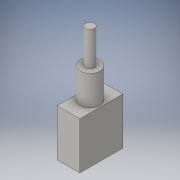
# Autodesk Inventor part: Switch
Saved by Autodesk Inventor 2016 (Build 200138000, 138)
## iProperties
Created: 2016-10-06
Part Number: Switch
Material: Generic
Document SubType Name: Modeling
Designer: sheehm
Density: 1 g/cm^3
Appearance: Default
Author: sheehm
Autodesk Inventor part; units mm, degrees
ref_plane "YZ Plane" through (0, 0, 0) normal (1, 0, 0) x (0, 1, 0)
ref_plane "XZ Plane" through (0, 0, 0) normal (0, 1, 0) x (-1, 0, 0)
ref_plane "XY Plane" through (0, 0, 0) normal (0, 0, 1) x (1, 0, 0)
sketch "Sketch1" plane through (0, 0, 0) normal (0, 1, 0) x (-1, 0, 0)
  line L0 (6.4234, 8.5987) -> (-0.2766, 8.5987)
  line L1 (-0.2766, 8.5987) -> (-0.2766, -4.1013)
  line L2 (-0.2766, -4.1013) -> (6.4234, -4.1013)
  line L3 (6.4234, -4.1013) -> (6.4234, 8.5987)
  point P0 (0, 0)
  dimension "d0" = 6.7
  dimension "d1" = 12.7
  constraints: 8 end point, 2 parallel, 1 horizontal, 1 perpendicular
  measures "d0" distance of L2.end L1.end
  measures "d1" distance of L1.end L0.end
extrude "Extrusion1" add sketch "Sketch1" along normal blind 13.9
sketch "Sketch2" plane through (0, 13.9, 0) normal (0, 1, 0) x (1, 0, 0)
  circle A0 centre (-3.0734, -2.2487) radius 2.93
  point P0 (0, 0)
  point P1 (-6.4234, -8.5987)
  point P2 (0.2766, -8.5987)
  point P3 (-6.4234, 4.1013)
  dimension "d4" = 5.86
  constraints: 1 centre point
  measures "d4" diameter of A0
extrude "Extrusion2" add sketch "Sketch2" along normal blind 8.8
sketch "Sketch3" plane through (-3.0734, 22.7, 2.2487) normal (0, 1, 0) x (1, 0, 0)
  circle A0 centre (0, 0) radius 1.3
  point P0 (3.0734, 2.2487)
  dimension "d7" = 2.6
  constraints: 1 centre point
  measures "d7" diameter of A0
extrude "Extrusion3" add sketch "Sketch3" along normal blind 10.1
body "Solid1"
